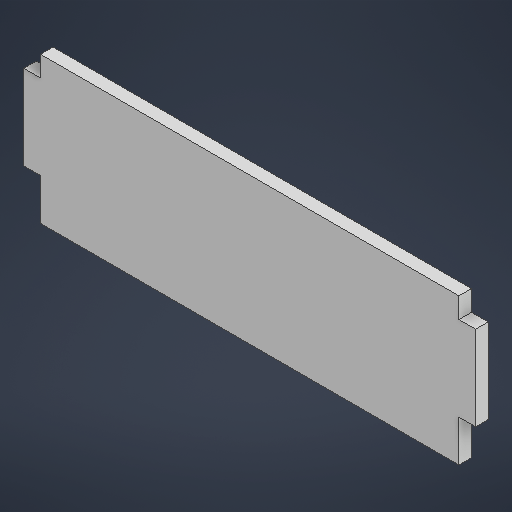
# Autodesk Inventor part: Battary_holder_part2
Saved by Autodesk Inventor 2027 (Build 310192000, 192)
## iProperties
Created: 2026-05-15
Part Number: Battary_holder_part2
Material: Generic
Document SubType Name: Modeling
Designer: alexy
Density: 1 g/cm^3
Appearance: Default
Author: alexy
Autodesk Inventor part; units mm, degrees
ref_plane "YZ Plane" through (0, 0, 0) normal (1, 0, 0) x (0, 1, 0)
ref_plane "XZ Plane" through (0, 0, 0) normal (0, 1, 0) x (-1, 0, 0)
ref_plane "XY Plane" through (0, 0, 0) normal (0, 0, 1) x (1, 0, 0)
sketch "Sketch1" plane through (0, 0, 0) normal (0, 0, 1) x (1, 0, 0)
  line L0 (0, 0) -> (100, 0)
  line L1 (100, 0) -> (100, 35)
  line L2 (100, 35) -> (0, 35)
  line L3 (0, 35) -> (0, 0)
  line L4 (104, 30.1) -> (100, 30.1)
  line L5 (100, 30.1) -> (100, 9.9)
  line L6 (100, 9.9) -> (104, 9.9)
  line L7 (104, 9.9) -> (104, 30.1)
  line L8 (104, 30.1) -> (100, 9.9) construction
  line L9 (100, 30.1) -> (104, 9.9) construction
  line L10 (-4, 30.1) -> (0, 30.1)
  line L11 (0, 30.1) -> (0, 9.9)
  line L12 (0, 9.9) -> (-4, 9.9)
  line L13 (-4, 9.9) -> (-4, 30.1)
  line L14 (-4, 30.1) -> (0, 9.9) construction
  line L15 (0, 30.1) -> (-4, 9.9) construction
  point P0 (102, 20)
  point P1 (-2, 20)
  point P2 (0, 30.1)
  point P3 (0, 30.1)
  point P4 (100, 30.1)
  point P5 (100, 25)
  point P6 (0, 25)
  dimension "d0" = 4
  dimension "d1" = 4
  dimension "d2" = 100
  dimension "d3" = 35
  dimension "d4" = 20.2
  dimension "d5" = 9.9
  constraints: 32 end point, 6 parallel, 4 midpoint, 3 horizontal, 3 perpendicular, 3 point on line, 2 horizontal alignment
  measures "d0" distance of L10.start L10.end
  measures "d1" distance of L4.start L4.end
  measures "d2" distance of L0.start L0.end
  measures "d3" distance of L0.end L1.end
  measures "d4" distance of L6.end L4.start
  measures "d5" distance from line of L0.end L6
extrude "Extrusion1" add sketch "Sketch1" along normal blind 3
body "Solid1"
